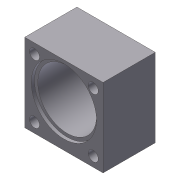
# Autodesk Inventor part: WheelBearingBlock
Saved by Autodesk Inventor 2012 (Build 160160000, 160)
## iProperties
Created: 2013-01-06
Part Number: WheelBearingBlock
Material: Aluminum-6061
Document SubType Name: Modeling
Designer: JesseK
Density: 2.71 g/cm^3
Mass: 49.3394 g
Surface Area: 92.106 cm^2
Volume: 18.2064 cm^3
Author: JesseK
Autodesk Inventor part; units mm, degrees
ref_plane "YZ Plane" through (0, 0, 0) normal (1, 0, 0) x (0, 1, 0)
ref_plane "XZ Plane" through (0, 0, 0) normal (0, 1, 0) x (-1, 0, 0)
ref_plane "XY Plane" through (0, 0, 0) normal (0, 0, 1) x (1, 0, 0)
sketch "Sketch1" plane through (0, 0, 0) normal (0, 0, 1) x (1, 0, 0)
  line L0 (-19.05, 19.05) -> (19.05, 19.05)
  line L1 (19.05, 19.05) -> (19.05, -19.05)
  line L2 (19.05, -19.05) -> (-19.05, -19.05)
  line L3 (-19.05, -19.05) -> (-19.05, 19.05)
  circle A0 centre (-14.2875, 14.2875) radius 2.4384
  circle A1 centre (14.2875, 14.2875) radius 2.4384
  circle A2 centre (14.2875, -14.2875) radius 2.4384
  circle A3 centre (-14.2875, -14.2875) radius 2.4384
  line L4 (-19.05, 15.875) -> (19.05, 15.875) construction
  line L5 (14.2875, 19.05) -> (14.2875, -19.05) construction
  line L6 (19.05, -12.7) -> (-19.05, -12.7) construction
  line L7 (-14.2875, -19.05) -> (-14.2875, 19.05) construction
  circle A4 centre (0, 1.5875) radius 14.2875
  point P0 (0, 0)
  dimension "d2" = 38.1
  dimension "d4" = 38.1
  dimension "d5" = 4.8768
  dimension "d6" = 4.7625
  dimension "d7" = 4.7625
  dimension "d8" = 4.7625
  dimension "d9" = 4.7625
  dimension "d10" = 4.7625
  dimension "d11" = 4.7625
  dimension "d12" = 4.7625
  dimension "d13" = 4.7625
  dimension "d22" = 19.05
  dimension "d23" = 6.35
  constraints: 16 end point, 8 point on line, 5 centre point, 4 tangent, 3 equal radius, 3 horizontal, 2 parallel, 2 vertical, 1 perpendicular
  measures "d2" distance of L0.end L1.end
  measures "d4" distance of L1.end L2.end
  measures "d5" diameter of A3
  measures "d6" distance from line of L2 A3.centre
  measures "d7" distance from line of L3 A3.centre
  measures "d8" distance from line of L3 A0.centre
  measures "d9" distance from line of L0 A0.centre
  measures "d10" distance from line of L0 A1.centre
  measures "d11" distance from line of L1 A1.centre
  measures "d12" distance from line of L1 A2.centre
  measures "d13" distance from line of L2 A2.centre
  measures "d22" distance from line of point (0, 0) L0
  measures "d23" distance between parallel lines of L2 L6
extrude "Extrusion4" add sketch "Sketch1" along normal blind 25.4
sketch "Sketch4" plane through (0, 0, 25.4) normal (0, 0, 1) x (1, 0, 0)
  circle A0 centre (0, 1.5875) radius 14.2875 projected
  circle A1 centre (0, 1.5875) radius 15.875
  circle A2 centre (0, 1.5875) radius 14.2875
  point P0 (0, 0)
  dimension "d26" = 1.5875
  constraints: 2 centre point, 2 coincident, 1 concentric
  measures "d26" radial gap between concentric circles of A1 A2
extrude "Extrusion5" cut sketch "Sketch4" against normal blind 1.5875
sketch "Sketch5" plane through (0, 0, 0) normal (0, 0, -1) x (-1, 0, 0)
  circle A0 centre (0, 1.5875) radius 14.2875 projected
  circle A1 centre (0, 1.5875) radius 15.875
  circle A2 centre (0, 1.5875) radius 14.2875
  point P0 (0, 0)
  dimension "d29" = 1.5875
  constraints: 2 centre point, 2 coincident, 1 concentric
  measures "d29" radial gap between concentric circles of A1 A2
extrude "Extrusion6" cut sketch "Sketch5" against normal blind 1.5875
body "Solid1"
